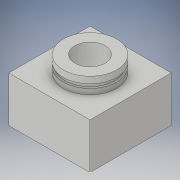
# Autodesk Inventor part: Part1
Saved by Autodesk Inventor 2018 (Build 220112000, 112)
## iProperties
Created: 2018-07-29
Part Number: Part1
Material: Generic
Document SubType Name: Modeling
Designer: BB-8
Density: 1 g/cm^3
Appearance: Default
Author: BB-8
Autodesk Inventor part; units mm, degrees
ref_plane "YZ Plane" through (0, 0, 0) normal (1, 0, 0) x (0, 1, 0)
ref_plane "XZ Plane" through (0, 0, 0) normal (0, 1, 0) x (-1, 0, 0)
ref_plane "XY Plane" through (0, 0, 0) normal (0, 0, 1) x (1, 0, 0)
sketch "Sketch1" plane through (0, 0, 0) normal (0, 1, 0) x (-1, 0, 0)
  point P0 (0, 0)
sketch "Sketch2" plane through (0, 0, 0) normal (0, 1, 0) x (-1, 0, 0)
  line L0 (0, 0) -> (76, 0)
  line L1 (76, 0) -> (76, -76)
  line L2 (76, -76) -> (0, -76)
  line L3 (0, -76) -> (0, 0)
  dimension "d3" = 76
  dimension "d4" = 76
  constraints: 8 end point, 2 parallel, 1 horizontal, 1 perpendicular
  measures "d3" distance of L1.end L2.end
  measures "d4" distance of L0.end L1.end
extrude "Extrusion1" add sketch "Sketch2" along normal blind 42.6
sketch "Sketch3" plane through (0, 42.6, 0) normal (0, 1, 0) x (1, 0, 0)
  circle A0 centre (-38, 38) radius 25
  point P0 (0, 0)
  dimension "d7" = 50
  constraints: 1 centre point
  measures "d7" diameter of A0
extrude "Extrusion2" add sketch "Sketch3" along normal blind 5.1
sketch "Sketch4" plane through (-38, 47.7, -38) normal (0, 1, 0) x (1, 0, 0)
  circle A0 centre (0, 0) radius 23
  point P0 (38, -38)
  dimension "d10" = 46
  constraints: 1 centre point
  measures "d10" diameter of A0
extrude "Extrusion3" add sketch "Sketch4" along normal blind 3.8
sketch "Sketch5" plane through (-38, 51.5, -38) normal (0, 1, 0) x (1, 0, 0)
  circle A0 centre (0, 0) radius 25
  point P0 (38, -38)
  constraints: 1 centre point
extrude "Extrusion4" add sketch "Sketch5" along normal blind 6.1
sketch "Sketch6" plane through (0, 0, 0) normal (0, -1, 0) x (1, 0, 0)
  circle A0 centre (-38, -38) radius 19
  point P0 (0, 0)
  dimension "d15" = 38
  constraints: 1 centre point
  measures "d15" diameter of A0
extrude "Extrusion5" cut sketch "Sketch6" against normal blind 8.1
sketch "Sketch7" plane through (-38, 8.1, -38) normal (0, -1, 0) x (1, 0, 0)
  circle A0 centre (0, 0) radius 14.2
  point P0 (38, 38)
  dimension "d18" = 28.4
  constraints: 1 centre point
  measures "d18" diameter of A0
extrude "Extrusion6" cut sketch "Sketch7" against normal blind 7
sketch "Sketch8" plane through (-38, 15.1, -38) normal (0, -1, 0) x (1, 0, 0)
  circle A0 centre (0, 0) radius 16.5
  point P0 (38, 38)
  dimension "d21" = 33
  constraints: 1 centre point
  measures "d21" diameter of A0
extrude "Extrusion7" cut sketch "Sketch8" against normal blind 12.5
sketch "Sketch9" plane through (-38, 57.6, -38) normal (0, 1, 0) x (1, 0, 0)
  circle A0 centre (0, 0) radius 14.2
  point P0 (38, -38)
  dimension "d24" = 28.4
  constraints: 1 centre point
  measures "d24" diameter of A0
extrude "Extrusion8" cut sketch "Sketch9" against normal blind 30
body "Solid1"
